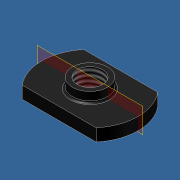
# Autodesk Inventor part: 20-081
Saved by Autodesk Inventor 2011 SP2 (Build 150309200, 309)
## iProperties
Shininess: 64.0
Length Units: 11269
Angle Units: 11279
Time Units: 11290
Mass Units: 11283
Length Display Precision: 5
Angle Display Precision: 2
Compacted: True
Part Number: 20-081
Document SubType Name: Modeling
Created: 2003-08-13
Designer: Graves
Material: Steel, Mild
Mass: 9.09856 g
Surface Area: 10.9587 cm^2
Volume: 1.15758 cm^3
Density: 7.86 g/cm^3
Density: 0.0
Volumn: 0.0
Area: 0.0
PropertySet Name: Model Information
Control State: 0
Master: False
Checked Out: False
Author: Graves
Autodesk Inventor part; units mm, degrees
ref_plane "YZ Plane" through (0, 0, 0) normal (1, 0, 0) x (0, 1, 0)
ref_plane "XY Plane" through (0, 0, 0) normal (0, 0, 1) x (1, 0, 0)
sketch "Sketch1" plane through (0, 0, 0) normal (0, 0, 1) x (1, 0, 0)
  line L0 (-9.6047, -8) -> (9.6047, -8)
  line L1 (9.6047, 8) -> (-9.6047, 8)
  line L2 (0, 11.2) -> (0, -11.2) projected
  line L3 (-17.5, 0) -> (17.5, 0) projected
  arc A0 (-9.6047, 8) -> (-9.6047, -8) centre (0, 0) ccw
  arc A1 (9.6047, -8) -> (9.6047, 8) centre (0, 0) ccw
  point P0 (0, 0)
  point P1 (0, -8)
  point P2 (12.5, 0)
  point P3 (-12.5, 0)
  dimension "d0" = 16
  dimension "d15" = 12.5
  dimension "d16" = 12.5
  dimension "d17" = 25
  dimension "d19" = 8
  constraints: 6 point on circle, 4 end point, 3 point on line, 2 centre point, 1 horizontal, 1 horizontal alignment, 1 midpoint, 1 parallel
  measures "d0" distance of L1.end L0.start
  measures "d15" radius of A1
  measures "d16" radius of A0
  measures "d17" distance of point (12.5, 0) point (-12.5, 0)
  measures "d19" distance between parallel lines of L1 L3
extrude "Extrusion1" add sketch "Sketch1" along normal blind 3.2
sketch "Sketch2" plane through (0, 0, 3.2) normal (0, 0, 1) x (1, 0, 0)
  line L0 (0, 11.2) -> (0, -11.2) projected
  line L1 (-17.5, 0) -> (17.5, 0) projected
  circle A0 centre (0, 0) radius 4.575
  dimension "d4" = 9.15
  constraints: 2 midpoint, 1 centre point
  measures "d4" diameter of A0
extrude "Extrusion2" add sketch "Sketch2" along normal blind 2.6
sketch "Sketch3" plane through (0, 0, 5.8) normal (0, 0, 1) x (1, 0, 0)
  circle A0 centre (0, 0) radius 4.575 projected
  constraints: 1 coincident
hole "Hole1" at (0, 0, 5.8) direction (0, 0, -1) diameter 6.647 end through all thread size "M8x1.25" class "6H" standard "ANSI Metric M Profile"
fillet "Fillet1" radius 0.5 1 edges at (-4.575, 0, 3.2)
body "Solid1"
